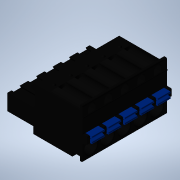
# Autodesk Inventor part: 8169608 5GD-1RR5,08-CLP-CBL
Saved by Autodesk Inventor 2021 (Build 250183000, 183)
## iProperties
Created: 2026-04-23
Part Number: 8169608 5GD-1RR5,08-CLP-CBL
Material: Generic
Catalog Web Link: www.3dfindit.com
Description: NEKM-C6 (p)-terminal strip
Vendor: FESTO
Document SubType Name: Modeling
Designer: psAdmin
Manufacturer: FESTO
Mass: 6.18347 g
Surface Area: 35.4957 cm^2
Volume: 6.18347 cm^3
Density: 1 g/cm^3
Appearance: PSOLRGB-80-80-80
Category: PARTsolutions
Company: FESTO
Title: 8169608 5GD-1RR5,08-CLP-CBL
Author: Cadenas PARTsolutions
Comments: terminal strip
PSOL_IDENT_0: {$CADENAS_DATA/23d-libs/festo/parts/n/nekm/parts/nekm_c6_parts.prj},200 {VTYP=3D},{NB=8169608 5GD-1R
PSOL_IDENT_1: R5,08-CLP-CBL},{LINA=8169608 5GD-1RR5,08-CLP-CBL},{NN=NEKM-C6 (p)},{DATE=26.08.2025 07:05:50},{GEOMD
PSOL_IDENT_2: ATE=26.08.2025 07:05:00},{VERSION=},{LINEID=150},{WBVAR=},{WBNUMERIC=}  {NB=8169608 5GD-1RR5,08-CLP-
PSOL_IDENT_3: CBL},{LINA=8169608 5GD-1RR5,08-CLP-CBL},{KT=DUMMY},{TNR=8169608},{TYP=5GD-1RR5,08-CLP-CBL},{VERS=2},
PSOL_IDENT_4: {N=5},{L=26.020},{L1=3.790}
NB: 8169608 5GD-1RR5,08-CLP-CBL
NN: NEKM-C6 (p)
NT: terminal strip
NBSYN: $TNR. $TYP.
LINA: 8169608 5GD-1RR5,08-CLP-CBL
CATALOG: Festo
TNR: 8169608
TYP: 5GD-1RR5,08-CLP-CBL
VERS: 2
N: 5
L: 26.02
L1: 3.79
SUPPLIER: FESTO
ARTICLENO: 8169608 5GD-1RR5,08-CLP-CBL
BOMINFO: 8169608 5GD-1RR5,08-CLP-CBL
CREATOR: CADENAS GmbH
Autodesk Inventor part; units mm, degrees
sketch "Sketch_1" plane through (0, 0, 0) normal (0, 0, 1) x (1, 0, 0)
  line L0 (0, 6) -> (0, -7.5)
  line L1 (0, -7.5) -> (14.43, -7.5)
  arc A0 (14.43, -7.5) -> (14.73, -7.2) centre (14.43, -7.2) ccw
  line L2 (14.73, -7.2) -> (14.73, 4.1)
  arc A1 (14.73, 4.1) -> (14.73, 4.5) centre (14.73, 4.3) ccw
  line L3 (14.73, 4.5) -> (14.73, 7.2)
  arc A2 (14.73, 7.2) -> (14.43, 7.5) centre (14.43, 7.2) ccw
  line L4 (14.43, 7.5) -> (13.93, 7.5)
  line L5 (13.93, 7.5) -> (13.93, 6)
  line L6 (13.93, 6) -> (0, 6)
  constraints: 14 end point, 6 point on circle, 3 centre point
extrude "Extrusion1" add sketch "Sketch_1" along normal mid plane 26.02
sketch "Sketch_2" plane through (0, 0, 13.01) normal (0, 0, 1) x (1, 0, 0)
  line L0 (14.73, 0.2) -> (14.73, -2.856)
  arc A0 (14.9274, -2.5741) -> (14.73, -2.856) centre (15.03, -2.856) ccw
  line L1 (14.9274, -2.5741) -> (16.0326, -2.1718)
  arc A1 (16.0326, -2.1718) -> (16.23, -1.8899) centre (15.93, -1.8899) ccw
  line L2 (16.23, -1.8899) -> (16.23, -0.3)
  arc A2 (16.23, -0.3) -> (15.93, 0) centre (15.93, -0.3) ccw
  line L3 (15.93, 0) -> (14.93, 0)
  arc A3 (14.73, 0.2) -> (14.93, 0) centre (14.93, 0.2) ccw
  constraints: 8 end point, 8 point on circle, 4 centre point
extrude "Extrusion2" add sketch "Sketch_2" against normal blind 0.8
pattern_linear "Rectangular Pattern1" count 2 spacing 25.22 along (0, 0, -1) of "Extrusion2"
sketch "Sketch_4" plane through (0, 0, 8.11) normal (0, 0, 1) x (1, 0, 0)
  line L0 (14.73, 0.2) -> (14.73, -2.756)
  arc A0 (14.9274, -2.4741) -> (14.73, -2.756) centre (15.03, -2.756) ccw
  line L1 (14.9274, -2.4741) -> (16.0326, -2.0718)
  arc A1 (16.0326, -2.0718) -> (16.23, -1.7899) centre (15.93, -1.7899) ccw
  line L2 (16.23, -1.7899) -> (16.23, -0.3)
  arc A2 (16.23, -0.3) -> (15.93, 0) centre (15.93, -0.3) ccw
  line L3 (15.93, 0) -> (14.93, 0)
  arc A3 (14.73, 0.2) -> (14.93, 0) centre (14.93, 0.2) ccw
  constraints: 8 end point, 8 point on circle, 4 centre point
extrude "Extrusion3" add sketch "Sketch_4" against normal blind 0.98
pattern_linear "Rectangular Pattern2" count 4 spacing 5.08 along (0, 0, -1) of "Extrusion3"
sketch "Sketch_6" plane through (0, 0, 12.11) normal (0, 0, 1) x (1, 0, 0)
  line L0 (14.73, -2.075) -> (16.6, -2.075)
  arc A0 (16.6, -2.075) -> (16.8, -1.875) centre (16.6, -1.875) ccw
  line L1 (16.8, -1.875) -> (16.8, -1.7601)
  arc A1 (16.8, -1.7601) -> (16.6041, -1.516) centre (16.55, -1.7601) ccw
  line L2 (16.6041, -1.516) -> (15.9359, -1.3679)
  arc A2 (15.9359, -0.7821) -> (15.9359, -1.3679) centre (16.0008, -1.075) ccw
  line L3 (15.9359, -0.7821) -> (16.6041, -0.634)
  arc A3 (16.6041, -0.634) -> (16.8, -0.3899) centre (16.55, -0.3899) ccw
  line L4 (16.8, -0.3899) -> (16.8, -0.275)
  arc A4 (16.8, -0.275) -> (16.6, -0.075) centre (16.6, -0.275) ccw
  line L5 (16.6, -0.075) -> (14.73, -0.075)
  line L6 (14.73, -0.075) -> (14.73, -2.075)
  constraints: 14 end point, 10 point on circle, 5 centre point
extrude "Extrusion4" add sketch "Sketch_6" against normal blind 3.9
pattern_linear "Rectangular Pattern3" count 5 spacing 5.08 along (0, 0, -1) of "Extrusion4"
sketch "Sketch_8" plane through (0, -4.65, 0) normal (0, 1, 0) x (1, 0, 0)
  line L0 (14.73, -10.36) -> (11.73, -10.36)
  line L1 (11.73, -10.36) -> (11.73, -8.36)
  line L2 (11.73, -8.36) -> (14.53, -8.36)
  arc A0 (14.53, -8.36) -> (14.73, -8.16) centre (14.53, -8.16) ccw
  line L3 (14.73, -8.16) -> (14.73, -10.36)
  line L4 (14.73, -10.36) -> (11.73, -10.36)
  constraints: 10 end point, 2 point on circle, 1 centre point
revolve "Revolution1" cut sketch "Sketch_8" angle 360 about axis through (14.73, -4.65, 10.36) along (1, 0, 0)
pattern_linear "Rectangular Pattern4" count 5 spacing 5.08 along (0, 0, -1) of "Revolution1"
sketch "Sketch_10" plane through (13.93, 0, 0) normal (1, 0, 0) x (0, 0, -1)
  line L0 (-12.4513, 6) -> (-7.8687, 6)
  arc A0 (-7.8687, 6) -> (-12.4513, 6) centre (-10.16, 5) ccw
  constraints: 2 end point, 2 point on circle, 1 centre point
extrude "Extrusion5" add sketch "Sketch_10" against normal blind 9.7
pattern_linear "Rectangular Pattern5" count 5 spacing 5.08 along (0, 0, -1) of "Extrusion5"
sketch "Sketch_12" plane through (0, 0, 0) normal (0, 0, 1) x (1, 0, 0)
  line L0 (2, 7.5) -> (2, 6)
  line L1 (2, 6) -> (4.23, 6)
  line L2 (4.23, 6) -> (5.73, 7.5)
  line L3 (5.73, 7.5) -> (2, 7.5)
  constraints: 8 end point
extrude "Extrusion6" cut sketch "Sketch_12" along normal mid plane 26.02
sketch "Sketch_13" plane through (14.73, 0, 0) normal (1, 0, 0) x (0, 0, -1)
  line L0 (-11.335, 5.775) -> (-11.335, 4.6)
  line L1 (-11.335, 4.6) -> (-8.985, 4.6)
  line L2 (-8.985, 4.6) -> (-8.985, 5.775)
  arc A0 (-8.985, 5.775) -> (-11.335, 5.775) centre (-10.16, 5.775) ccw
  constraints: 6 end point, 2 point on circle, 1 centre point
extrude "Extrusion7" cut sketch "Sketch_13" against normal blind 9.325
pattern_linear "Rectangular Pattern6" count 5 spacing 5.08 along (0, 0, -1) of "Extrusion7"
sketch "Sketch_15" plane through (0, 7.5, 0) normal (0, 1, 0) x (1, 0, 0)
  arc A0 (5.405, -8.985) -> (5.405, -11.335) centre (5.405, -10.16) ccw
  line L0 (5.405, -11.335) -> (6.58, -11.335)
  line L1 (6.58, -11.335) -> (6.58, -8.985)
  line L2 (6.58, -8.985) -> (5.405, -8.985)
  constraints: 6 end point, 2 point on circle, 1 centre point
extrude "Extrusion8" cut sketch "Sketch_15" against normal blind 2.9
pattern_linear "Rectangular Pattern7" count 5 spacing 5.08 along (0, 0, -1) of "Extrusion8"
sketch "Sketch_17" plane through (3.13, 0, 0) normal (1, 0, 0) x (0, 0, -1)
  line L0 (-10.16, 6) -> (-10.16, 6.3)
  arc A0 (-9.71, 6) -> (-10.16, 6.3) centre (-10.1683, 5.8001) ccw
  line L1 (-9.71, 6) -> (-10.16, 6)
  line L2 (-10.16, 6) -> (-10.16, 6.3)
  constraints: 6 end point, 2 point on circle, 1 centre point
revolve "Revolution2" add sketch "Sketch_17" angle 360 about axis through (3.13, 6, 10.16) along (0, -1, 0)
pattern_linear "Rectangular Pattern8" count 5 spacing 5.08 along (0, 0, -1) of "Revolution2"
sketch "Sketch_25" plane through (0, 0, 0) normal (0, 0, 1) x (1, 0, 0)
  line L0 (-0.5, -0.795) -> (-0.5, -7.5)
  line L1 (-0.5, -7.5) -> (0, -7.5)
  line L2 (0, -7.5) -> (0, 0.071)
  line L3 (0, 0.071) -> (-0.5, -0.795)
  constraints: 8 end point
extrude "Extrusion9" add sketch "Sketch_25" along normal mid plane 26.02
sketch "Sketch_41" plane through (-0.5, 0, 0) normal (1, 0, 0) x (0, 0, -1)
  line L0 (-12.7, -5.71) -> (-12.2807, -5.71)
  arc A0 (-12.2807, -5.71) -> (-8.0393, -5.71) centre (-10.16, -3.71) ccw
  line L1 (-8.0393, -5.71) -> (-7.2007, -5.71)
  arc A1 (-7.2007, -5.71) -> (-2.9593, -5.71) centre (-5.08, -3.71) ccw
  line L2 (-2.9593, -5.71) -> (-2.1207, -5.71)
  arc A2 (-2.1207, -5.71) -> (2.1207, -5.71) centre (0, -3.71) ccw
  line L3 (2.1207, -5.71) -> (2.9593, -5.71)
  arc A3 (2.9593, -5.71) -> (7.2007, -5.71) centre (5.08, -3.71) ccw
  line L4 (7.2007, -5.71) -> (8.0393, -5.71)
  arc A4 (8.0393, -5.71) -> (12.2807, -5.71) centre (10.16, -3.71) ccw
  line L5 (12.2807, -5.71) -> (12.7, -5.71)
  line L6 (12.7, -5.71) -> (12.7, -0.795)
  line L7 (12.7, -0.795) -> (11.417, -0.795)
  line L8 (11.417, -0.795) -> (11.8096, -1.475)
  line L9 (11.8096, -1.475) -> (8.5134, -1.475)
  line L10 (8.5134, -1.475) -> (8.906, -0.795)
  line L11 (8.906, -0.795) -> (6.337, -0.795)
  line L12 (6.337, -0.795) -> (6.7296, -1.475)
  line L13 (6.7296, -1.475) -> (3.4334, -1.475)
  line L14 (3.4334, -1.475) -> (3.826, -0.795)
  line L15 (3.826, -0.795) -> (1.257, -0.795)
  line L16 (1.257, -0.795) -> (1.6496, -1.475)
  line L17 (1.6496, -1.475) -> (-1.6466, -1.475)
  line L18 (-1.6466, -1.475) -> (-1.254, -0.795)
  line L19 (-1.254, -0.795) -> (-3.823, -0.795)
  line L20 (-3.823, -0.795) -> (-3.4304, -1.475)
  line L21 (-3.4304, -1.475) -> (-6.7266, -1.475)
  line L22 (-6.7266, -1.475) -> (-6.334, -0.795)
  line L23 (-6.334, -0.795) -> (-8.903, -0.795)
  line L24 (-8.903, -0.795) -> (-8.5104, -1.475)
  line L25 (-8.5104, -1.475) -> (-11.8066, -1.475)
  line L26 (-11.8066, -1.475) -> (-11.414, -0.795)
  line L27 (-11.414, -0.795) -> (-12.7, -0.795)
  line L28 (-12.7, -0.795) -> (-12.7, -5.71)
  constraints: 58 end point, 10 point on circle, 5 centre point
extrude "Extrusion10" add sketch "Sketch_41" against normal blind 8.3
sketch "Sketch13" plane through (-8.8, 0, 0) normal (-1, 0, 0) x (0, 0, 1)
  point P0 (10.16, -3.71)
hole "Hole1" at (-8.8, -3.71, 10.16) direction (1, 0, 0) diameter 1.4 depth 2 counterbore diameter 2.8 counterbore depth 1
pattern_linear "Rectangular Pattern9" count 5 spacing 5.08 along (0, 0, -1) of "Hole1"
sketch "Sketch_30" plane through (0, 0, 9.22) normal (0, 0, 1) x (1, 0, 0)
  arc A0 (-4.9014, 1.2616) -> (-4.86, 0.947) centre (-4.76, 1.1202) ccw
  line L0 (-4.86, 0.947) -> (-4.1642, 0.5453)
  arc A1 (-4.1642, 0.5453) -> (-3.8021, 0.5929) centre (-4.0142, 0.8051) ccw
  line L1 (-3.8021, 0.5929) -> (-3.53, 0.865)
  line L2 (-3.53, 0.865) -> (-0.3256, 1.0049)
  arc A2 (-0.3, 0.406) -> (-0.3256, 1.0049) centre (-0.3, 0.706) ccw
  arc A3 (-0.3, 0.406) -> (-0.5, 0.206) centre (-0.3, 0.206) ccw
  line L3 (-0.5, 0.206) -> (-0.5, -1)
  line L4 (-0.5, -1) -> (0.5, -1)
  line L5 (0.5, -1) -> (0.5, 3.3534)
  line L6 (0.5, 3.3534) -> (0, 3.3534)
  arc A4 (-0.2325, 3.0611) -> (0, 3.3534) centre (-0.3, 3.3534) ccw
  line L7 (-0.2325, 3.0611) -> (-3.7536, 2.2482)
  arc A5 (-3.7536, 2.2482) -> (-4.1152, 2.0478) centre (-3.5849, 1.5174) ccw
  line L8 (-4.1152, 2.0478) -> (-4.9014, 1.2616)
  constraints: 18 end point, 12 point on circle, 6 centre point
extrude "Extrusion11" add sketch "Sketch_30" against normal blind 1.6
sketch "Sketch_31" plane through (0, 0, -9.22) normal (0, 0, 1) x (1, 0, 0)
  arc A0 (-4.9014, 1.2616) -> (-4.86, 0.947) centre (-4.76, 1.1202) ccw
  line L0 (-4.86, 0.947) -> (-4.1642, 0.5453)
  arc A1 (-4.1642, 0.5453) -> (-3.8021, 0.5929) centre (-4.0142, 0.8051) ccw
  line L1 (-3.8021, 0.5929) -> (-3.53, 0.865)
  line L2 (-3.53, 0.865) -> (-0.3256, 1.0049)
  arc A2 (-0.3, 0.406) -> (-0.3256, 1.0049) centre (-0.3, 0.706) ccw
  arc A3 (-0.3, 0.406) -> (-0.5, 0.206) centre (-0.3, 0.206) ccw
  line L3 (-0.5, 0.206) -> (-0.5, -1)
  line L4 (-0.5, -1) -> (0.5, -1)
  line L5 (0.5, -1) -> (0.5, 3.3534)
  line L6 (0.5, 3.3534) -> (0, 3.3534)
  arc A4 (-0.2325, 3.0611) -> (0, 3.3534) centre (-0.3, 3.3534) ccw
  line L7 (-0.2325, 3.0611) -> (-3.7536, 2.2482)
  arc A5 (-3.7536, 2.2482) -> (-4.1152, 2.0478) centre (-3.5849, 1.5174) ccw
  line L8 (-4.1152, 2.0478) -> (-4.9014, 1.2616)
  constraints: 18 end point, 12 point on circle, 6 centre point
extrude "Extrusion12" add sketch "Sketch_31" along normal blind 1.6
sketch "Sketch_42" plane through (11.58, 0, 0) normal (1, 0, 0) x (0, 0, -1)
  line L0 (-13.01, -8.25) -> (13.01, -8.25)
  line L1 (13.01, -8.25) -> (13.01, -6.25)
  line L2 (13.01, -6.25) -> (12.3185, -6.25)
  arc A0 (7.6015, -6.25) -> (12.3185, -6.25) centre (9.96, -4.65) ccw
  line L3 (7.6015, -6.25) -> (7.2385, -6.25)
  arc A1 (2.5215, -6.25) -> (7.2385, -6.25) centre (4.88, -4.65) ccw
  line L4 (2.5215, -6.25) -> (2.1585, -6.25)
  arc A2 (-2.5585, -6.25) -> (2.1585, -6.25) centre (-0.2, -4.65) ccw
  line L5 (-2.5585, -6.25) -> (-2.9215, -6.25)
  arc A3 (-7.6385, -6.25) -> (-2.9215, -6.25) centre (-5.28, -4.65) ccw
  line L6 (-7.6385, -6.25) -> (-8.0015, -6.25)
  arc A4 (-12.7185, -6.25) -> (-8.0015, -6.25) centre (-10.36, -4.65) ccw
  line L7 (-12.7185, -6.25) -> (-13.01, -6.25)
  line L8 (-13.01, -6.25) -> (-13.01, -8.25)
  constraints: 18 end point, 10 point on circle, 5 centre point
extrude "Extrusion13" cut sketch "Sketch_42" along normal blind 2.35
ref_plane "ANBAU_XY" through (0, 0, 0) normal (0, 1, 0) x (1, 0, 0)
ref_plane "ANBAU_YZ" through (0, 0, 0) normal (1, 0, 0) x (0, 0, -1)
ref_plane "ANBAU_ZX" through (0, 0, 0) normal (0, 0, -1) x (0, 1, 0)
ref_plane "CP1_XY" through (-0.5, -3.71, 0) normal (1, 0, 0) x (0, 0, -1)
ref_plane "CP1_YZ" through (-0.5, -3.71, 0) normal (0, 0, -1) x (0, 1, 0)
ref_plane "CP1_ZX" through (-0.5, -3.71, 0) normal (0, 1, 0) x (1, 0, 0)
ref_plane "ECP_1_XY" through (2.73, -4.65, 10.36) normal (1, 0, 0) x (0, 0, -1)
ref_plane "ECP_1_YZ" through (2.73, -4.65, 10.36) normal (0, 0, -1) x (0, 1, 0)
ref_plane "ECP_1_ZX" through (2.73, -4.65, 10.36) normal (0, 1, 0) x (1, 0, 0)
ref_plane "ECP_2_XY" through (2.73, -4.65, 5.28) normal (1, 0, 0) x (0, 0, -1)
ref_plane "ECP_2_YZ" through (2.73, -4.65, 5.28) normal (0, 0, -1) x (0, 1, 0)
ref_plane "ECP_2_ZX" through (2.73, -4.65, 5.28) normal (0, 1, 0) x (1, 0, 0)
ref_plane "ECP_3_XY" through (2.73, -4.65, 0.2) normal (1, 0, 0) x (0, 0, -1)
ref_plane "ECP_3_YZ" through (2.73, -4.65, 0.2) normal (0, 0, -1) x (0, 1, 0)
ref_plane "ECP_3_ZX" through (2.73, -4.65, 0.2) normal (0, 1, 0) x (1, 0, 0)
ref_plane "ECP_4_XY" through (2.73, -4.65, -4.88) normal (1, 0, 0) x (0, 0, -1)
ref_plane "ECP_4_YZ" through (2.73, -4.65, -4.88) normal (0, 0, -1) x (0, 1, 0)
ref_plane "ECP_4_ZX" through (2.73, -4.65, -4.88) normal (0, 1, 0) x (1, 0, 0)
ref_plane "ECP_5_XY" through (2.73, -4.65, -9.96) normal (1, 0, 0) x (0, 0, -1)
ref_plane "ECP_5_YZ" through (2.73, -4.65, -9.96) normal (0, 0, -1) x (0, 1, 0)
ref_plane "ECP_5_ZX" through (2.73, -4.65, -9.96) normal (0, 1, 0) x (1, 0, 0)
ref_plane "MD_XY" through (-8.8, -3.71, 10.16) normal (-1, 0, 0) x (0, 0, -1)
ref_plane "MD_YZ" through (-8.8, -3.71, 10.16) normal (0, 0, -1) x (0, -1, 0)
ref_plane "MD_ZX" through (-8.8, -3.71, 10.16) normal (0, -1, 0) x (-1, 0, 0)
ref_plane "OP_XY" through (-8.8, 7.5, -13.01) normal (1, 0, 0) x (0, 0, 1)
ref_plane "OP_YZ" through (-8.8, 7.5, -13.01) normal (0, 0, 1) x (0, -1, 0)
ref_plane "OP_ZX" through (-8.8, 7.5, -13.01) normal (0, -1, 0) x (1, 0, 0)
body "Solid1"
